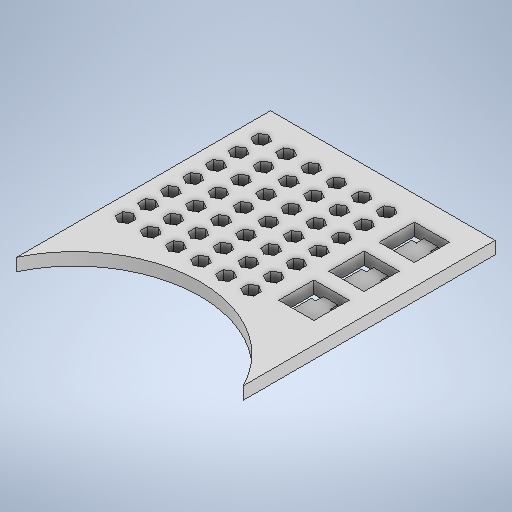
# Autodesk Inventor part: pokrywka
Saved by Autodesk Inventor 2025.2 (Build 292293000, 293)
## iProperties
Created: 2025-08-28
Part Number: pokrywka
Material: Ogólny
Document SubType Name: Modeling
Designer: IGOR
Density: 1 g/cm^3
Appearance: Domyślna
Author: IGOR
## iProperties of the stored document pokrywka_Drukowanie 3D.ipt
Created: 2025-08-28
Part Number: pokrywka_Drukowanie 3D
Material: Ogólny
Document SubType Name: Modeling
Designer: IGOR
Density: 1 g/cm^3
Appearance: Domyślna
Author: IGOR
Autodesk Inventor part; units mm, degrees
ref_plane "YZ Plane" through (0, 0, 0) normal (1, 0, 0) x (0, 1, 0)
ref_plane "XZ Plane" through (0, 0, 0) normal (0, 1, 0) x (-1, 0, 0)
ref_plane "XY Plane" through (0, 0, 0) normal (0, 0, 1) x (1, 0, 0)
sketch "Szkic1" plane through (0, 0, 0) normal (0, 1, 0) x (-1, 0, 0)
  line L0 (45.0348, 50.4958) -> (45.0348, -50.7281)
  line L1 (-44.4428, -50.7328) -> (45.0348, -50.7328)
  line L2 (45.0348, -50.7328) -> (45.0348, 50.4958)
  line L3 (-44.8833, 50.4957) -> (-44.4428, 50.4957)
  line L4 (-44.4428, 50.4957) -> (-44.4428, -50.7328)
  arc A0 (-44.8833, 50.4957) -> (45.0348, 50.2743) centre (0.1296, 72.2636) ccw
  arc A1 (-39.9428, 32.1405) -> (40.5348, 32.4757) centre (0.1296, 72.2636) ccw
  line L5 (-39.9428, -46.2328) -> (40.5348, -46.2328)
  line L6 (40.5348, -46.2328) -> (40.5348, 32.4757)
  line L7 (-39.9428, 32.1405) -> (-39.9428, -46.2328)
  point P0 (0, 0)
  point P1 (40.5348, -6.8786)
  point P2 (45.0348, 50.2743)
  point P3 (-44.4428, 49.6074)
  dimension "d0" = 4.5
  dimension "d1" = 4.5
  dimension "d2" = 4.5
  dimension "d3" = 6.7067
  dimension "d4" = 4.5
  dimension "d5" = 50
  constraints: 16 end point, 4 point on circle, 3 parallel, 2 centre point, 2 horizontal, 2 perpendicular, 1 coincident, 1 midpoint, 1 point on line
  measures "d0" distance from line of point (40.535, -6.879) L0
  measures "d1" distance between parallel lines of L4 L7
  measures "d2" distance between parallel lines of L1 L5
  measures "d3" radial gap between concentric circles of A1 A0
  measures "d4" distance between parallel lines of L2 L6
  measures "d5" radius of A0
extrude "Wyciągnięcie proste1" add sketch "Szkic1" along normal blind 5 contours L0 L2 L1 L4 A0 | A1 L6 L5 L7
sketch "Szkic2" plane through (0, 5, 0) normal (0, 1, 0) x (1, 0, 0)
  line L0 (22, 41) -> (36, 41)
  line L1 (36, 41) -> (36, 27)
  line L2 (36, 27) -> (22, 27)
  line L3 (22, 27) -> (22, 41)
  line L4 (22, 41) -> (36, 27) construction
  line L5 (36, 41) -> (22, 27) construction
  line L6 (24, 30) -> (34, 30)
  line L7 (34, 30) -> (34, 38)
  line L8 (34, 38) -> (24, 38)
  line L9 (24, 38) -> (24, 30)
  line L10 (24, 30) -> (34, 38) construction
  line L11 (34, 30) -> (24, 38) construction
  line L12 (44.4428, -49.6074) -> (44.4428, 50.7328) projected
  line L13 (44.4428, 50.7328) -> (44.4428, -49.6074)
  line L14 (44.4428, -49.6074) -> (-46.0859, -49.6074)
  line L15 (36, 21) -> (36, 7)
  line L16 (34, 10) -> (34, 18)
  line L17 (24, 10) -> (34, 10)
  line L18 (36, 7) -> (22, 7)
  line L19 (22, 7) -> (22, 21)
  line L20 (24, 18) -> (24, 10)
  line L21 (34, 18) -> (24, 18)
  line L22 (22, 21) -> (36, 21)
  line L23 (36, 1) -> (36, -13)
  line L24 (34, -10) -> (34, -2)
  line L25 (24, -10) -> (34, -10)
  line L26 (36, -13) -> (22, -13)
  line L27 (22, -13) -> (22, 1)
  line L28 (24, -2) -> (24, -10)
  line L29 (34, -2) -> (24, -2)
  line L30 (22, 1) -> (36, 1)
  line L31 (16, 41) -> (16, 27)
  line L32 (14, 30) -> (14, 38)
  line L33 (4, 30) -> (14, 30)
  line L34 (16, 27) -> (2, 27)
  line L35 (2, 27) -> (2, 41)
  line L36 (4, 38) -> (4, 30)
  line L37 (14, 38) -> (4, 38)
  line L38 (2, 41) -> (16, 41)
  line L39 (16, 21) -> (16, 7)
  line L40 (14, 10) -> (14, 18)
  line L41 (4, 10) -> (14, 10)
  line L42 (16, 7) -> (2, 7)
  line L43 (2, 7) -> (2, 21)
  line L44 (4, 18) -> (4, 10)
  line L45 (14, 18) -> (4, 18)
  line L46 (2, 21) -> (16, 21)
  line L47 (16, 1) -> (16, -13)
  line L48 (14, -10) -> (14, -2)
  line L49 (4, -10) -> (14, -10)
  line L50 (16, -13) -> (2, -13)
  line L51 (2, -13) -> (2, 1)
  line L52 (4, -2) -> (4, -10)
  line L53 (14, -2) -> (4, -2)
  line L54 (2, 1) -> (16, 1)
  line L55 (31.6, 41) -> (25.8, 41)
  line L56 (25.8, 41) -> (25.8, 38)
  line L57 (25.8, 38) -> (31.6, 38)
  line L58 (31.6, 38) -> (31.6, 41)
  line L59 (31.6, 30) -> (25.8, 30)
  line L60 (25.8, 30) -> (25.8, 27)
  line L61 (25.8, 27) -> (31.6, 27)
  line L62 (31.6, 27) -> (31.6, 30)
  line L63 (31.6, 18) -> (25.8, 18)
  line L64 (25.8, 18) -> (25.8, 21)
  line L65 (25.8, 21) -> (31.6, 21)
  line L66 (31.6, 21) -> (31.6, 18)
  line L67 (31.6, 10) -> (25.8, 10)
  line L68 (25.8, 10) -> (25.8, 7)
  line L69 (25.8, 7) -> (31.6, 7)
  line L70 (31.6, 7) -> (31.6, 10)
  line L71 (31.6, -2) -> (25.8, -2)
  line L72 (25.8, -2) -> (25.8, 1)
  line L73 (25.8, 1) -> (31.6, 1)
  line L74 (31.6, 1) -> (31.6, -2)
  line L75 (31.6, -10) -> (25.8, -10)
  line L76 (25.8, -10) -> (25.8, -13)
  line L77 (25.8, -13) -> (31.6, -13)
  line L78 (31.6, -13) -> (31.6, -10)
  point P0 (29, 34)
  dimension "d8" = 14
  dimension "d9" = 14
  dimension "d12" = 20
  dimension "d15" = 20
  constraints: 156 end point, 17 equal length, 17 point on line, 9 horizontal, 9 perpendicular, 4 midpoint, 1 vertical, 80 other
  measures "d8" distance of L1.end L2.end
  measures "d9" distance of L0.end L1.end
  measures "d12" distance of L0.end L15.start
  measures "d15" distance of L0.end L31.start
extrude "Wyciągnięcie proste2" cut sketch "Szkic2" against normal blind 3.8 contours L8 L7 L6 L9 | L21 L16 L17 L20 | L29 L24 L25 L28
extrude "Wyciągnięcie proste3" cut sketch "Szkic2" against normal blind 3.8 contours L0 L58 L8 L56 | L60 L6 L62 L2 | L66 L21 L64 L22 | L18 L68 L17 L70 | L74 L29 L72 L30 | L26 L76 L25 L78
extrude "Wyciągnięcie proste4" cut sketch "Szkic2" against normal through all contours L0 L56 L8 L9 L6 L60 L2 L3 | L0 L1 L2 L62 L6 L7 L8 L58 | L15 L18 L70 L17 L16 L21 L66 L22 | L64 L21 L20 L17 L68 L18 L19 L22 | L23 L26 L78 L25 L24 L29 L74 L30 | L72 L29 L28 L25 L76 L26 L27 L30
sketch "Szkic3" plane through (0, 5, 0) normal (0, 1, 0) x (1, 0, 0)
  line L0 (13, 36) -> (10.4019, 37.5)
  line L1 (10.4019, 37.5) -> (10.4019, 40.5)
  line L2 (10.4019, 40.5) -> (13, 42)
  line L3 (13, 42) -> (15.5981, 40.5)
  line L4 (15.5981, 40.5) -> (15.5981, 37.5)
  line L5 (15.5981, 37.5) -> (13, 36)
  line L6 (44.4428, 50.7328) -> (-45.0348, 50.7328) projected
  line L7 (18.0419, 50.7328) -> (18.0419, -53)
  line L8 (18.0419, -53) -> (-41.8483, -53)
  line L9 (15.5981, 28.5) -> (13, 27)
  line L10 (15.5981, 31.5) -> (15.5981, 28.5)
  line L11 (10.4019, 31.5) -> (13, 33)
  line L12 (10.4019, 28.5) -> (10.4019, 31.5)
  line L13 (13, 27) -> (10.4019, 28.5)
  line L14 (13, 33) -> (15.5981, 31.5)
  line L15 (15.5981, 19.5) -> (13, 18)
  line L16 (15.5981, 22.5) -> (15.5981, 19.5)
  line L17 (10.4019, 22.5) -> (13, 24)
  line L18 (10.4019, 19.5) -> (10.4019, 22.5)
  line L19 (13, 18) -> (10.4019, 19.5)
  line L20 (13, 24) -> (15.5981, 22.5)
  line L21 (15.5981, 10.5) -> (13, 9)
  line L22 (15.5981, 13.5) -> (15.5981, 10.5)
  line L23 (10.4019, 13.5) -> (13, 15)
  line L24 (10.4019, 10.5) -> (10.4019, 13.5)
  line L25 (13, 9) -> (10.4019, 10.5)
  line L26 (13, 15) -> (15.5981, 13.5)
  line L27 (15.5981, 1.5) -> (13, 0)
  line L28 (15.5981, 4.5) -> (15.5981, 1.5)
  line L29 (10.4019, 4.5) -> (13, 6)
  line L30 (10.4019, 1.5) -> (10.4019, 4.5)
  line L31 (13, 0) -> (10.4019, 1.5)
  line L32 (13, 6) -> (15.5981, 4.5)
  line L33 (15.5981, -7.5) -> (13, -9)
  line L34 (15.5981, -4.5) -> (15.5981, -7.5)
  line L35 (10.4019, -4.5) -> (13, -3)
  line L36 (10.4019, -7.5) -> (10.4019, -4.5)
  line L37 (13, -9) -> (10.4019, -7.5)
  line L38 (13, -3) -> (15.5981, -4.5)
  line L39 (15.5981, -16.5) -> (13, -18)
  line L40 (15.5981, -13.5) -> (15.5981, -16.5)
  line L41 (10.4019, -13.5) -> (13, -12)
  line L42 (10.4019, -16.5) -> (10.4019, -13.5)
  line L43 (13, -18) -> (10.4019, -16.5)
  line L44 (13, -12) -> (15.5981, -13.5)
  line L45 (5.5981, 37.5) -> (3, 36)
  line L46 (5.5981, 40.5) -> (5.5981, 37.5)
  line L47 (0.4019, 40.5) -> (3, 42)
  line L48 (0.4019, 37.5) -> (0.4019, 40.5)
  line L49 (3, 36) -> (0.4019, 37.5)
  line L50 (3, 42) -> (5.5981, 40.5)
  line L51 (5.5981, 28.5) -> (3, 27)
  line L52 (5.5981, 31.5) -> (5.5981, 28.5)
  line L53 (0.4019, 31.5) -> (3, 33)
  line L54 (0.4019, 28.5) -> (0.4019, 31.5)
  line L55 (3, 27) -> (0.4019, 28.5)
  line L56 (3, 33) -> (5.5981, 31.5)
  line L57 (5.5981, 19.5) -> (3, 18)
  line L58 (5.5981, 22.5) -> (5.5981, 19.5)
  line L59 (0.4019, 22.5) -> (3, 24)
  line L60 (0.4019, 19.5) -> (0.4019, 22.5)
  line L61 (3, 18) -> (0.4019, 19.5)
  line L62 (3, 24) -> (5.5981, 22.5)
  line L63 (5.5981, 10.5) -> (3, 9)
  line L64 (5.5981, 13.5) -> (5.5981, 10.5)
  line L65 (0.4019, 13.5) -> (3, 15)
  line L66 (0.4019, 10.5) -> (0.4019, 13.5)
  line L67 (3, 9) -> (0.4019, 10.5)
  line L68 (3, 15) -> (5.5981, 13.5)
  line L69 (5.5981, 1.5) -> (3, 0)
  line L70 (5.5981, 4.5) -> (5.5981, 1.5)
  line L71 (0.4019, 4.5) -> (3, 6)
  line L72 (0.4019, 1.5) -> (0.4019, 4.5)
  line L73 (3, 0) -> (0.4019, 1.5)
  line L74 (3, 6) -> (5.5981, 4.5)
  line L75 (5.5981, -7.5) -> (3, -9)
  line L76 (5.5981, -4.5) -> (5.5981, -7.5)
  line L77 (0.4019, -4.5) -> (3, -3)
  line L78 (0.4019, -7.5) -> (0.4019, -4.5)
  line L79 (3, -9) -> (0.4019, -7.5)
  line L80 (3, -3) -> (5.5981, -4.5)
  line L81 (5.5981, -16.5) -> (3, -18)
  line L82 (5.5981, -13.5) -> (5.5981, -16.5)
  line L83 (0.4019, -13.5) -> (3, -12)
  line L84 (0.4019, -16.5) -> (0.4019, -13.5)
  line L85 (3, -18) -> (0.4019, -16.5)
  line L86 (3, -12) -> (5.5981, -13.5)
  line L87 (-4.4019, 37.5) -> (-7, 36)
  line L88 (-4.4019, 40.5) -> (-4.4019, 37.5)
  line L89 (-9.5981, 40.5) -> (-7, 42)
  line L90 (-9.5981, 37.5) -> (-9.5981, 40.5)
  line L91 (-7, 36) -> (-9.5981, 37.5)
  line L92 (-7, 42) -> (-4.4019, 40.5)
  line L93 (-4.4019, 28.5) -> (-7, 27)
  line L94 (-4.4019, 31.5) -> (-4.4019, 28.5)
  line L95 (-9.5981, 31.5) -> (-7, 33)
  line L96 (-9.5981, 28.5) -> (-9.5981, 31.5)
  line L97 (-7, 27) -> (-9.5981, 28.5)
  line L98 (-7, 33) -> (-4.4019, 31.5)
  line L99 (-4.4019, 19.5) -> (-7, 18)
  line L100 (-4.4019, 22.5) -> (-4.4019, 19.5)
  line L101 (-9.5981, 22.5) -> (-7, 24)
  line L102 (-9.5981, 19.5) -> (-9.5981, 22.5)
  line L103 (-7, 18) -> (-9.5981, 19.5)
  line L104 (-7, 24) -> (-4.4019, 22.5)
  line L105 (-4.4019, 10.5) -> (-7, 9)
  line L106 (-4.4019, 13.5) -> (-4.4019, 10.5)
  line L107 (-9.5981, 13.5) -> (-7, 15)
  line L108 (-9.5981, 10.5) -> (-9.5981, 13.5)
  line L109 (-7, 9) -> (-9.5981, 10.5)
  line L110 (-7, 15) -> (-4.4019, 13.5)
  line L111 (-4.4019, 1.5) -> (-7, 0)
  line L112 (-4.4019, 4.5) -> (-4.4019, 1.5)
  line L113 (-9.5981, 4.5) -> (-7, 6)
  line L114 (-9.5981, 1.5) -> (-9.5981, 4.5)
  line L115 (-7, 0) -> (-9.5981, 1.5)
  line L116 (-7, 6) -> (-4.4019, 4.5)
  line L117 (-4.4019, -7.5) -> (-7, -9)
  line L118 (-4.4019, -4.5) -> (-4.4019, -7.5)
  line L119 (-9.5981, -4.5) -> (-7, -3)
  line L120 (-9.5981, -7.5) -> (-9.5981, -4.5)
  line L121 (-7, -9) -> (-9.5981, -7.5)
  line L122 (-7, -3) -> (-4.4019, -4.5)
  line L123 (-4.4019, -16.5) -> (-7, -18)
  line L124 (-4.4019, -13.5) -> (-4.4019, -16.5)
  line L125 (-9.5981, -13.5) -> (-7, -12)
  line L126 (-9.5981, -16.5) -> (-9.5981, -13.5)
  line L127 (-7, -18) -> (-9.5981, -16.5)
  line L128 (-7, -12) -> (-4.4019, -13.5)
  line L129 (-14.4019, 37.5) -> (-17, 36)
  line L130 (-14.4019, 40.5) -> (-14.4019, 37.5)
  line L131 (-19.5981, 40.5) -> (-17, 42)
  line L132 (-19.5981, 37.5) -> (-19.5981, 40.5)
  line L133 (-17, 36) -> (-19.5981, 37.5)
  line L134 (-17, 42) -> (-14.4019, 40.5)
  line L135 (-14.4019, 28.5) -> (-17, 27)
  line L136 (-14.4019, 31.5) -> (-14.4019, 28.5)
  line L137 (-19.5981, 31.5) -> (-17, 33)
  line L138 (-19.5981, 28.5) -> (-19.5981, 31.5)
  line L139 (-17, 27) -> (-19.5981, 28.5)
  line L140 (-17, 33) -> (-14.4019, 31.5)
  line L141 (-14.4019, 19.5) -> (-17, 18)
  line L142 (-14.4019, 22.5) -> (-14.4019, 19.5)
  line L143 (-19.5981, 22.5) -> (-17, 24)
  line L144 (-19.5981, 19.5) -> (-19.5981, 22.5)
  line L145 (-17, 18) -> (-19.5981, 19.5)
  line L146 (-17, 24) -> (-14.4019, 22.5)
  line L147 (-14.4019, 10.5) -> (-17, 9)
  line L148 (-14.4019, 13.5) -> (-14.4019, 10.5)
  line L149 (-19.5981, 13.5) -> (-17, 15)
  line L150 (-19.5981, 10.5) -> (-19.5981, 13.5)
  line L151 (-17, 9) -> (-19.5981, 10.5)
  line L152 (-17, 15) -> (-14.4019, 13.5)
  line L153 (-14.4019, 1.5) -> (-17, 0)
  line L154 (-14.4019, 4.5) -> (-14.4019, 1.5)
  line L155 (-19.5981, 4.5) -> (-17, 6)
  line L156 (-19.5981, 1.5) -> (-19.5981, 4.5)
  line L157 (-17, 0) -> (-19.5981, 1.5)
  line L158 (-17, 6) -> (-14.4019, 4.5)
  line L159 (-14.4019, -7.5) -> (-17, -9)
  line L160 (-14.4019, -4.5) -> (-14.4019, -7.5)
  line L161 (-19.5981, -4.5) -> (-17, -3)
  line L162 (-19.5981, -7.5) -> (-19.5981, -4.5)
  line L163 (-17, -9) -> (-19.5981, -7.5)
  line L164 (-17, -3) -> (-14.4019, -4.5)
  line L165 (-14.4019, -16.5) -> (-17, -18)
  line L166 (-14.4019, -13.5) -> (-14.4019, -16.5)
  line L167 (-19.5981, -13.5) -> (-17, -12)
  line L168 (-19.5981, -16.5) -> (-19.5981, -13.5)
  line L169 (-17, -18) -> (-19.5981, -16.5)
  line L170 (-17, -12) -> (-14.4019, -13.5)
  line L171 (-24.4019, 37.5) -> (-27, 36)
  line L172 (-24.4019, 40.5) -> (-24.4019, 37.5)
  line L173 (-29.5981, 40.5) -> (-27, 42)
  line L174 (-29.5981, 37.5) -> (-29.5981, 40.5)
  line L175 (-27, 36) -> (-29.5981, 37.5)
  line L176 (-27, 42) -> (-24.4019, 40.5)
  line L177 (-24.4019, 28.5) -> (-27, 27)
  line L178 (-24.4019, 31.5) -> (-24.4019, 28.5)
  line L179 (-29.5981, 31.5) -> (-27, 33)
  line L180 (-29.5981, 28.5) -> (-29.5981, 31.5)
  line L181 (-27, 27) -> (-29.5981, 28.5)
  line L182 (-27, 33) -> (-24.4019, 31.5)
  line L183 (-24.4019, 19.5) -> (-27, 18)
  line L184 (-24.4019, 22.5) -> (-24.4019, 19.5)
  line L185 (-29.5981, 22.5) -> (-27, 24)
  line L186 (-29.5981, 19.5) -> (-29.5981, 22.5)
  line L187 (-27, 18) -> (-29.5981, 19.5)
  line L188 (-27, 24) -> (-24.4019, 22.5)
  line L189 (-24.4019, 10.5) -> (-27, 9)
  line L190 (-24.4019, 13.5) -> (-24.4019, 10.5)
  line L191 (-29.5981, 13.5) -> (-27, 15)
  line L192 (-29.5981, 10.5) -> (-29.5981, 13.5)
  line L193 (-27, 9) -> (-29.5981, 10.5)
  line L194 (-27, 15) -> (-24.4019, 13.5)
  line L195 (-24.4019, 1.5) -> (-27, 0)
  line L196 (-24.4019, 4.5) -> (-24.4019, 1.5)
  line L197 (-29.5981, 4.5) -> (-27, 6)
  line L198 (-29.5981, 1.5) -> (-29.5981, 4.5)
  line L199 (-27, 0) -> (-29.5981, 1.5)
  line L200 (-27, 6) -> (-24.4019, 4.5)
  line L201 (-24.4019, -7.5) -> (-27, -9)
  line L202 (-24.4019, -4.5) -> (-24.4019, -7.5)
  line L203 (-29.5981, -4.5) -> (-27, -3)
  line L204 (-29.5981, -7.5) -> (-29.5981, -4.5)
  line L205 (-27, -9) -> (-29.5981, -7.5)
  line L206 (-27, -3) -> (-24.4019, -4.5)
  line L207 (-24.4019, -16.5) -> (-27, -18)
  line L208 (-24.4019, -13.5) -> (-24.4019, -16.5)
  line L209 (-29.5981, -13.5) -> (-27, -12)
  line L210 (-29.5981, -16.5) -> (-29.5981, -13.5)
  line L211 (-27, -18) -> (-29.5981, -16.5)
  line L212 (-27, -12) -> (-24.4019, -13.5)
  line L213 (-34.4019, 37.5) -> (-37, 36)
  line L214 (-34.4019, 40.5) -> (-34.4019, 37.5)
  line L215 (-39.5981, 40.5) -> (-37, 42)
  line L216 (-39.5981, 37.5) -> (-39.5981, 40.5)
  line L217 (-37, 36) -> (-39.5981, 37.5)
  line L218 (-37, 42) -> (-34.4019, 40.5)
  line L219 (-34.4019, 28.5) -> (-37, 27)
  line L220 (-34.4019, 31.5) -> (-34.4019, 28.5)
  line L221 (-39.5981, 31.5) -> (-37, 33)
  line L222 (-39.5981, 28.5) -> (-39.5981, 31.5)
  line L223 (-37, 27) -> (-39.5981, 28.5)
  line L224 (-37, 33) -> (-34.4019, 31.5)
  line L225 (-34.4019, 19.5) -> (-37, 18)
  line L226 (-34.4019, 22.5) -> (-34.4019, 19.5)
  line L227 (-39.5981, 22.5) -> (-37, 24)
  line L228 (-39.5981, 19.5) -> (-39.5981, 22.5)
  line L229 (-37, 18) -> (-39.5981, 19.5)
  line L230 (-37, 24) -> (-34.4019, 22.5)
  line L231 (-34.4019, 10.5) -> (-37, 9)
  line L232 (-34.4019, 13.5) -> (-34.4019, 10.5)
  line L233 (-39.5981, 13.5) -> (-37, 15)
  line L234 (-39.5981, 10.5) -> (-39.5981, 13.5)
  line L235 (-37, 9) -> (-39.5981, 10.5)
  line L236 (-37, 15) -> (-34.4019, 13.5)
  line L237 (-34.4019, 1.5) -> (-37, 0)
  line L238 (-34.4019, 4.5) -> (-34.4019, 1.5)
  line L239 (-39.5981, 4.5) -> (-37, 6)
  line L240 (-39.5981, 1.5) -> (-39.5981, 4.5)
  line L241 (-37, 0) -> (-39.5981, 1.5)
  line L242 (-37, 6) -> (-34.4019, 4.5)
  line L243 (-34.4019, -7.5) -> (-37, -9)
  line L244 (-34.4019, -4.5) -> (-34.4019, -7.5)
  line L245 (-39.5981, -4.5) -> (-37, -3)
  line L246 (-39.5981, -7.5) -> (-39.5981, -4.5)
  line L247 (-37, -9) -> (-39.5981, -7.5)
  line L248 (-37, -3) -> (-34.4019, -4.5)
  line L249 (-34.4019, -16.5) -> (-37, -18)
  line L250 (-34.4019, -13.5) -> (-34.4019, -16.5)
  line L251 (-39.5981, -13.5) -> (-37, -12)
  line L252 (-39.5981, -16.5) -> (-39.5981, -13.5)
  line L253 (-37, -18) -> (-39.5981, -16.5)
  line L254 (-37, -12) -> (-34.4019, -13.5)
  point P0 (0, 0)
  point P1 (13, 39)
  dimension "d26" = 9
  dimension "d29" = 10
  constraints: 508 end point, 2 vertical, 1 horizontal, 1 perpendicular, 1 point on line, 505 other
  measures "d26" distance of L4.end L9.start
  measures "d29" distance of L4.end L45.start
extrude "Wyciągnięcie proste5" cut sketch "Szkic3" against normal through all
